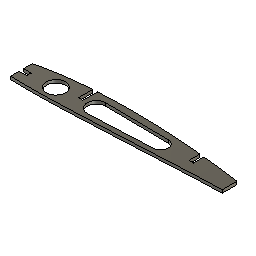
Ala_sola (Autodesk Fusion 360 design; units mm, degrees)
Autodesk Fusion 360 part; units mm, degrees
sketch "Sketch1" plane through (0, 0, -356.8897) normal (0, 0, -1) x (1, 0, 0)
  spline S0 degree 3 poles (-314.9041, -27.3143) (-316.3315, -27.2751) (-317.7488, -27.2348) (-319.1559, -27.1934) (-320.4817, -27.1544) (-321.8989, -27.1118) (-323.4076, -27.0655) (-325.0648, -27.0147) (-326.482, -26.9692) (-327.659, -26.9291) (-329.1964, -26.8766) (-330.6132, -26.8239) (-331.9096, -26.7707) (-333.2219, -26.7169) (-334.6383, -26.653) (-336.1588, -26.579) (-337.3657, -26.5203) (-338.7817, -26.4481) (-340.4069, -26.3625) (-340.9048, -26.3362) (-342.3207, -26.2608) (-344.6545, -26.1362) (-346.3871, -26.0437) (-347.803, -25.9687) (-348.9022, -25.9112) (-350.4533, -25.8302) (-351.8693, -25.7578) (-353.1502, -25.6942) (-354.3709, -25.6336) (-355.7871, -25.5655) (-357.3988, -25.49) (-357.8647, -25.4681) (-358.5729, -25.4351) (-359.5233, -25.3909) (-360.4753, -25.3466) (-361.1835, -25.3136) (-361.6478, -25.2918) (-363.3057, -25.2141) (-364.7219, -25.1456) (-365.8964, -25.0864) (-367.081, -25.0266) (-368.4969, -24.9521) (-370.1441, -24.8628) (-370.6018, -24.8379) (-371.3096, -24.7993) (-372.2678, -24.7469) (-373.1875, -24.6965) (-373.8954, -24.658) (-374.3914, -24.6312) (-375.1751, -24.589) (-375.883, -24.5515) (-376.5152, -24.5187) (-377.2155, -24.4825) (-377.9236, -24.447) (-378.6393, -24.4121) (-379.7568, -24.3578) (-381.1731, -24.2918) (-382.8883, -24.2142) (-383.038, -24.2074) (-383.7462, -24.1755) (-385.0129, -24.1185) (-385.8708, -24.0798) (-386.579, -24.0477) (-387.1375, -24.0222) (-388.4675, -23.9613) (-389.8838, -23.8946) (-391.3864, -23.8221) (-392.4634, -23.7701) (-393.8796, -23.7008) (-395.6349, -23.6141) (-397.743, -23.51) (-399.1591, -23.4403) (-399.8833, -23.405) (-401.4759, -23.3273) (-402.8922, -23.2596) (-404.1321, -23.2021) (-405.6617, -23.1311) (-407.0782, -23.0681) (-408.3815, -23.0132) (-409.7162, -22.957) (-411.1329, -22.901) (-412.6317, -22.8453) (-413.9257, -22.7972) (-415.3427, -22.7469) (-416.8826, -22.6944) (-418.2291, -22.6484) (-419.6462, -22.6016) (-421.1339, -22.5538) (-422.7685, -22.5013) (-424.1858, -22.4583) (-425.3855, -22.4248) (-427.0005, -22.3797) (-428.418, -22.3467) (-429.6379, -22.3256) (-430.9059, -22.3038) (-432.3237, -22.2887) (-433.8912, -22.2804) (-434.4617, -22.2774) (-435.1706, -22.2747) (-436.018, -22.2724) (-436.7269, -22.2704) (-437.4359, -22.2685) (-438.1448, -22.2667) (-438.154, -22.2666) (-438.5085, -22.2655) (-439.2082, -22.2633) (-439.6355, -22.262) (-439.99, -22.2609) (-440.2716, -22.2601) (-441.1017, -22.2579) (-441.8106, -22.2568) (-442.3984, -22.2568) (-443.1776, -22.2569) (-443.8865, -22.2589) (-444.5252, -22.2629) (-445.2443, -22.2674) (-445.9532, -22.2751) (-446.6518, -22.2858) (-448.0829, -22.3077) (-449.5003, -22.3423) (-450.9041, -22.3898) knots 0.19390624 0.19390624 0.19390624 0.19390624 0.20388368 0.20388368 0.20388368 0.21386113 0.21386113 0.21386113 0.22383858 0.22383858 0.22383858 0.23381602 0.23381602 0.23381602 0.24379347 0.24379347 0.24379347 0.25377092 0.25377092 0.25377092 0.26374837 0.26374837 0.26374837 0.27372581 0.27372581 0.27372581 0.28370326 0.28370326 0.28370326 0.29368071 0.29368071 0.29368071 0.29866943 0.29866943 0.29866943 0.30365815 0.30365815 0.30365815 0.3136356 0.3136356 0.3136356 0.32361305 0.32361305 0.32361305 0.32860177 0.32860177 0.32860177 0.3335905 0.3335905 0.3335905 0.33857922 0.33857922 0.33857922 0.34356794 0.34356794 0.34356794 0.35354539 0.35354539 0.35354539 0.35853411 0.35853411 0.35853411 0.36352284 0.36352284 0.36352284 0.37350028 0.37350028 0.37350028 0.38347773 0.38347773 0.38347773 0.39345518 0.39345518 0.39345518 0.40343263 0.40343263 0.40343263 0.41341007 0.41341007 0.41341007 0.42338752 0.42338752 0.42338752 0.43336497 0.43336497 0.43336497 0.44334241 0.44334241 0.44334241 0.45331986 0.45331986 0.45331986 0.46329731 0.46329731 0.46329731 0.47327476 0.47327476 0.47327476 0.47826348 0.47826348 0.47826348 0.4832522 0.4832522 0.4832522 0.48574656 0.48574656 0.48574656 0.48824093 0.48824093 0.48824093 0.49322965 0.49322965 0.49322965 0.49821837 0.49821837 0.49821837 0.5032071 0.5032071 0.5032071 0.51318454 0.51318454 0.51318454 0.51318454
  line L0 (-450.9041, -22.3898) -> (-450.9041, -28.1007)
  line L1 (-450.9041, -28.1007) -> (-445.9041, -28.1007)
  line L2 (-445.9041, -28.1007) -> (-445.9041, -31.1007)
  line L3 (-445.9041, -31.1007) -> (-450.9041, -31.1007)
  line L4 (-450.9041, -31.1007) -> (-450.9041, -36.8116)
  spline S1 degree 3 poles (-450.9041, -36.8116) (-450.2054, -36.9947) (-449.4894, -37.1753) (-448.7562, -37.3534) (-448.0397, -37.5274) (-447.3208, -37.6955) (-446.5992, -37.8577) (-445.2244, -38.1667) (-443.7786, -38.4677) (-442.262, -38.7606) (-440.8373, -39.0357) (-439.3839, -39.297) (-437.9016, -39.5444) (-436.4787, -39.7819) (-435.0193, -40.0079) (-433.5236, -40.2223) (-432.0873, -40.4282) (-430.6235, -40.6232) (-429.1321, -40.8074) (-427.6736, -40.9874) (-426.2064, -41.1548) (-424.7304, -41.3095) (-423.301, -41.4593) (-421.831, -41.6002) (-420.3203, -41.7323) (-418.863, -41.8597) (-417.3909, -41.9773) (-415.9041, -42.0849) knots 0.007053 0.007053 0.007053 0.007053 0.012249 0.012249 0.012249 0.017445 0.017445 0.017445 0.027837 0.027837 0.027837 0.038229 0.038229 0.038229 0.048621 0.048621 0.048621 0.059013 0.059013 0.059013 0.069404 0.069404 0.069404 0.079796 0.079796 0.079796 0.090188 0.090188 0.090188 0.090188
  line L5 (-415.9041, -42.0849) -> (-415.9041, -32.5613)
  line L6 (-415.9041, -32.5613) -> (-412.9041, -32.5613)
  line L7 (-412.9041, -32.5613) -> (-412.9041, -42.2874)
  spline S2 degree 3 poles (-412.9041, -42.2874) (-410.0329, -42.4672) (-407.1159, -42.6103) (-404.1532, -42.7167) (-402.6996, -42.7689) (-401.24, -42.812) (-399.7744, -42.846) (-398.3395, -42.8793) (-396.8794, -42.9043) (-395.3942, -42.9212) (-393.945, -42.9377) (-392.4848, -42.9462) (-391.0135, -42.9467) (-389.5879, -42.9472) (-388.1277, -42.9402) (-386.6327, -42.9256) (-383.6825, -42.8969) (-380.7625, -42.8411) (-377.8728, -42.7582) (-374.9901, -42.6756) (-372.0717, -42.5646) (-369.1177, -42.4253) (-366.2195, -42.2887) (-363.3036, -42.1258) (-360.3698, -41.9367) (-358.7322, -41.8312) (-357.0673, -41.716) (-355.3751, -41.591) (-353.6901, -41.4666) (-352.0263, -41.3363) (-350.3838, -41.2002) (-347.9215, -40.996) (-345.4283, -40.7717) (-342.9041, -40.5272) knots 0.835586 0.835586 0.835586 0.835586 0.856138 0.856138 0.856138 0.866414 0.866414 0.866414 0.87669 0.87669 0.87669 0.886966 0.886966 0.886966 0.897242 0.897242 0.897242 0.917793 0.917793 0.917793 0.938345 0.938345 0.938345 0.958897 0.958897 0.958897 0.97064 0.97064 0.97064 0.982384 0.982384 0.982384 1 1 1 1
  line L8 (-342.9041, -40.5272) -> (-342.9041, -33.3089)
  line L9 (-342.9041, -33.3089) -> (-339.9041, -33.3089)
  line L10 (-339.9041, -33.3089) -> (-339.9041, -40.2289)
  spline S3 degree 3 poles (-339.9041, -40.2289) (-337.8749, -40.0221) (-335.7879, -39.7995) (-333.643, -39.5611) (-331.4764, -39.3202) (-329.3915, -39.0785) (-327.3883, -38.836) (-325.2965, -38.5827) (-323.2143, -38.3187) (-321.1416, -38.044) (-319.1073, -37.7744) (-317.0281, -37.4876) (-314.9041, -37.1837) knots 0.769436 0.769436 0.769436 0.769436 0.784206 0.784206 0.784206 0.798975 0.798975 0.798975 0.813745 0.813745 0.813745 0.828515 0.828515 0.828515 0.828515
  line L11 (-314.9041, -37.1837) -> (-314.9041, -27.3143)
  circle A0 centre (-429.337, -31.1007) radius 6.3498
  arc A1 (-403.3199, -26.4196) -> (-403.9041, -38.7308) centre (-403.9041, -32.5613) ccw
  line L12 (-403.3199, -26.4196) -> (-361.8196, -28.389)
  arc A2 (-361.8196, -38.2288) -> (-361.8196, -28.389) centre (-361.8196, -33.3089) ccw
  line L13 (-361.8196, -38.2288) -> (-403.9041, -38.7308)
extrude "Extrude1" add sketch "Sketch1" against normal blind 2
sketch "Sketch2" plane through (0, 0, -356.8897) normal (0, 0, -1) x (1, 0, 0)
  circle A0 centre (-429.337, -31.1007) radius 6.3498
  arc A1 (-403.3199, -26.4196) -> (-403.9041, -38.7308) centre (-403.9041, -32.5613) ccw
  line L0 (-403.3199, -26.4196) -> (-361.8196, -28.389)
  arc A2 (-361.8196, -38.2288) -> (-361.8196, -28.389) centre (-361.8196, -33.3089) ccw
  line L1 (-361.8196, -38.2288) -> (-403.9041, -38.7308)
  line L2 (-314.9041, -37.1837) -> (-314.9041, -27.3143)
  spline S0 degree 3 poles (-314.9041, -27.3143) (-316.3315, -27.2751) (-317.7488, -27.2348) (-319.1559, -27.1934) (-320.4817, -27.1544) (-321.8989, -27.1118) (-323.4076, -27.0655) (-325.0648, -27.0147) (-326.482, -26.9692) (-327.659, -26.9291) (-329.1964, -26.8766) (-330.6132, -26.8239) (-331.9096, -26.7707) (-333.2219, -26.7169) (-334.6383, -26.653) (-336.1588, -26.579) (-337.3657, -26.5203) (-338.7817, -26.4481) (-340.4069, -26.3625) (-340.9048, -26.3362) (-342.3207, -26.2608) (-344.6545, -26.1362) (-346.3871, -26.0437) (-347.803, -25.9687) (-348.9022, -25.9112) (-350.4533, -25.8302) (-351.8693, -25.7578) (-353.1502, -25.6942) (-354.3709, -25.6336) (-355.7871, -25.5655) (-357.3988, -25.49) (-357.8647, -25.4681) (-358.5729, -25.4351) (-359.5233, -25.3909) (-360.4753, -25.3466) (-361.1835, -25.3136) (-361.6478, -25.2918) (-363.3057, -25.2141) (-364.7219, -25.1456) (-365.8964, -25.0864) (-367.081, -25.0266) (-368.4969, -24.9521) (-370.1441, -24.8628) (-370.6018, -24.8379) (-371.3096, -24.7993) (-372.2678, -24.7469) (-373.1875, -24.6965) (-373.8954, -24.658) (-374.3914, -24.6312) (-375.1751, -24.589) (-375.883, -24.5515) (-376.5152, -24.5187) (-377.2155, -24.4825) (-377.9236, -24.447) (-378.6393, -24.4121) (-379.7568, -24.3578) (-381.1731, -24.2918) (-382.8883, -24.2142) (-383.038, -24.2074) (-383.7462, -24.1755) (-385.0129, -24.1185) (-385.8708, -24.0798) (-386.579, -24.0477) (-387.1375, -24.0222) (-388.4675, -23.9613) (-389.8838, -23.8946) (-391.3864, -23.8221) (-392.4634, -23.7701) (-393.8796, -23.7008) (-395.6349, -23.6141) (-397.743, -23.51) (-399.1591, -23.4403) (-399.8833, -23.405) (-401.4759, -23.3273) (-402.8922, -23.2596) (-404.1321, -23.2021) (-405.6617, -23.1311) (-407.0782, -23.0681) (-408.3815, -23.0132) (-409.7162, -22.957) (-411.1329, -22.901) (-412.6317, -22.8453) (-413.9257, -22.7972) (-415.3427, -22.7469) (-416.8826, -22.6944) (-418.2291, -22.6484) (-419.6462, -22.6016) (-421.1339, -22.5538) (-422.7685, -22.5013) (-424.1858, -22.4583) (-425.3855, -22.4248) (-427.0005, -22.3797) (-428.418, -22.3467) (-429.6379, -22.3256) (-430.9059, -22.3038) (-432.3237, -22.2887) (-433.8912, -22.2804) (-434.4617, -22.2774) (-435.1706, -22.2747) (-436.018, -22.2724) (-436.7269, -22.2704) (-437.4359, -22.2685) (-438.1448, -22.2667) (-438.154, -22.2666) (-438.5085, -22.2655) (-439.2082, -22.2633) (-439.6355, -22.262) (-439.99, -22.2609) (-440.2716, -22.2601) (-441.1017, -22.2579) (-441.8106, -22.2568) (-442.3984, -22.2568) (-443.1776, -22.2569) (-443.8865, -22.2589) (-444.5252, -22.2629) (-445.2443, -22.2674) (-445.9532, -22.2751) (-446.6518, -22.2858) (-448.0829, -22.3077) (-449.5003, -22.3423) (-450.9041, -22.3898) knots 0.19390624 0.19390624 0.19390624 0.19390624 0.20388368 0.20388368 0.20388368 0.21386113 0.21386113 0.21386113 0.22383858 0.22383858 0.22383858 0.23381602 0.23381602 0.23381602 0.24379347 0.24379347 0.24379347 0.25377092 0.25377092 0.25377092 0.26374837 0.26374837 0.26374837 0.27372581 0.27372581 0.27372581 0.28370326 0.28370326 0.28370326 0.29368071 0.29368071 0.29368071 0.29866943 0.29866943 0.29866943 0.30365815 0.30365815 0.30365815 0.3136356 0.3136356 0.3136356 0.32361305 0.32361305 0.32361305 0.32860177 0.32860177 0.32860177 0.3335905 0.3335905 0.3335905 0.33857922 0.33857922 0.33857922 0.34356794 0.34356794 0.34356794 0.35354539 0.35354539 0.35354539 0.35853411 0.35853411 0.35853411 0.36352284 0.36352284 0.36352284 0.37350028 0.37350028 0.37350028 0.38347773 0.38347773 0.38347773 0.39345518 0.39345518 0.39345518 0.40343263 0.40343263 0.40343263 0.41341007 0.41341007 0.41341007 0.42338752 0.42338752 0.42338752 0.43336497 0.43336497 0.43336497 0.44334241 0.44334241 0.44334241 0.45331986 0.45331986 0.45331986 0.46329731 0.46329731 0.46329731 0.47327476 0.47327476 0.47327476 0.47826348 0.47826348 0.47826348 0.4832522 0.4832522 0.4832522 0.48574656 0.48574656 0.48574656 0.48824093 0.48824093 0.48824093 0.49322965 0.49322965 0.49322965 0.49821837 0.49821837 0.49821837 0.5032071 0.5032071 0.5032071 0.51318454 0.51318454 0.51318454 0.51318454
  line L3 (-450.9041, -22.3898) -> (-450.9041, -28.1007)
  line L4 (-450.9041, -28.1007) -> (-445.9041, -28.1007)
  line L5 (-445.9041, -28.1007) -> (-445.9041, -31.1007)
  line L6 (-445.9041, -31.1007) -> (-450.9041, -31.1007)
  line L7 (-450.9041, -31.1007) -> (-450.9041, -36.8116)
  spline S1 degree 3 poles (-450.9041, -36.8116) (-450.2054, -36.9947) (-449.4894, -37.1753) (-448.7562, -37.3534) (-448.0397, -37.5274) (-447.3208, -37.6955) (-446.5992, -37.8577) (-445.2244, -38.1667) (-443.7786, -38.4677) (-442.262, -38.7606) (-440.8373, -39.0357) (-439.3839, -39.297) (-437.9016, -39.5444) (-436.4787, -39.7819) (-435.0193, -40.0079) (-433.5236, -40.2223) (-432.0873, -40.4282) (-430.6235, -40.6232) (-429.1321, -40.8074) (-427.6736, -40.9874) (-426.2064, -41.1548) (-424.7304, -41.3095) (-423.301, -41.4593) (-421.831, -41.6002) (-420.3203, -41.7323) (-418.863, -41.8597) (-417.3909, -41.9773) (-415.9041, -42.0849) knots 0.007053 0.007053 0.007053 0.007053 0.012249 0.012249 0.012249 0.017445 0.017445 0.017445 0.027837 0.027837 0.027837 0.038229 0.038229 0.038229 0.048621 0.048621 0.048621 0.059013 0.059013 0.059013 0.069404 0.069404 0.069404 0.079796 0.079796 0.079796 0.090188 0.090188 0.090188 0.090188
  line L8 (-415.9041, -42.0849) -> (-415.9041, -32.5613)
  line L9 (-415.9041, -32.5613) -> (-412.9041, -32.5613)
  line L10 (-412.9041, -32.5613) -> (-412.9041, -42.2874)
  spline S2 degree 3 poles (-412.9041, -42.2874) (-410.0329, -42.4672) (-407.1159, -42.6103) (-404.1532, -42.7167) (-402.6996, -42.7689) (-401.24, -42.812) (-399.7744, -42.846) (-398.3395, -42.8793) (-396.8794, -42.9043) (-395.3942, -42.9212) (-393.945, -42.9377) (-392.4848, -42.9462) (-391.0135, -42.9467) (-389.5879, -42.9472) (-388.1277, -42.9402) (-386.6327, -42.9256) (-383.6825, -42.8969) (-380.7625, -42.8411) (-377.8728, -42.7582) (-374.9901, -42.6756) (-372.0717, -42.5646) (-369.1177, -42.4253) (-366.2195, -42.2887) (-363.3036, -42.1258) (-360.3698, -41.9367) (-358.7322, -41.8312) (-357.0673, -41.716) (-355.3751, -41.591) (-353.6901, -41.4666) (-352.0263, -41.3363) (-350.3838, -41.2002) (-347.9215, -40.996) (-345.4283, -40.7717) (-342.9041, -40.5272) knots 0.835586 0.835586 0.835586 0.835586 0.856138 0.856138 0.856138 0.866414 0.866414 0.866414 0.87669 0.87669 0.87669 0.886966 0.886966 0.886966 0.897242 0.897242 0.897242 0.917793 0.917793 0.917793 0.938345 0.938345 0.938345 0.958897 0.958897 0.958897 0.97064 0.97064 0.97064 0.982384 0.982384 0.982384 1 1 1 1
  line L11 (-342.9041, -40.5272) -> (-342.9041, -33.3089)
  line L12 (-342.9041, -33.3089) -> (-339.9041, -33.3089)
  line L13 (-339.9041, -33.3089) -> (-339.9041, -40.2289)
  spline S3 degree 3 poles (-339.9041, -40.2289) (-337.8749, -40.0221) (-335.7879, -39.7995) (-333.643, -39.5611) (-331.4764, -39.3202) (-329.3915, -39.0785) (-327.3883, -38.836) (-325.2965, -38.5827) (-323.2143, -38.3187) (-321.1416, -38.044) (-319.1073, -37.7744) (-317.0281, -37.4876) (-314.9041, -37.1837) knots 0.769436 0.769436 0.769436 0.769436 0.784206 0.784206 0.784206 0.798975 0.798975 0.798975 0.813745 0.813745 0.813745 0.828515 0.828515 0.828515 0.828515
  line L14 (-412.9041, -32.5613) -> (-415.9041, -32.5613)
  line L15 (-415.9041, -32.5613) -> (-415.9041, -47.9137)
  line L16 (-415.9041, -47.9137) -> (-412.9041, -47.9137)
  line L17 (-412.9041, -47.9137) -> (-412.9041, -32.5613)
  line L18 (-342.9041, -33.3089) -> (-339.9041, -33.3089)
  line L19 (-339.9041, -33.3089) -> (-339.9041, -44.8961)
  line L20 (-339.9041, -44.8961) -> (-342.9041, -44.8961)
  line L21 (-342.9041, -44.8961) -> (-342.9041, -33.3089)
  line L22 (-445.9041, -28.1007) -> (-458.839, -28.1007)
  line L23 (-458.839, -28.1007) -> (-458.839, -31.1007)
  line L24 (-458.839, -31.1007) -> (-445.9041, -31.1007)
  line L25 (-445.9041, -31.1007) -> (-445.9041, -28.1007)
  circle A3 centre (-429.337, -31.1007) radius 6.3498
  constraint horizontal L14
  constraint vertical L15
  constraint horizontal L16
  constraint vertical L17
  constraint coincident L9.end L10.start
  constraint horizontal L18
  constraint vertical L19
  constraint horizontal L20
  constraint vertical L21
  constraint coincident L11.end L12.start
  constraint coincident L8.end L9.start
  constraint horizontal L22
  constraint vertical L23
  constraint horizontal L24
  constraint vertical L25
  constraint coincident L4.end L5.start
sketch "Sketch3" plane through (0, 0, -356.8897) normal (0, 0, -1) x (1, 0, 0)
  circle A0 centre (-429.337, -31.1007) radius 6.3498
  arc A1 (-403.3199, -26.4196) -> (-403.9041, -38.7308) centre (-403.9041, -32.5613) ccw
  line L0 (-403.3199, -26.4196) -> (-361.8196, -28.389)
  arc A2 (-361.8196, -38.2288) -> (-361.8196, -28.389) centre (-361.8196, -33.3089) ccw
  line L1 (-361.8196, -38.2288) -> (-403.9041, -38.7308)
  line L2 (-314.9041, -37.1837) -> (-314.9041, -27.3143)
  spline S0 degree 3 poles (-314.9041, -27.3143) (-316.3315, -27.2751) (-317.7488, -27.2348) (-319.1559, -27.1934) (-320.4817, -27.1544) (-321.8989, -27.1118) (-323.4076, -27.0655) (-325.0648, -27.0147) (-326.482, -26.9692) (-327.659, -26.9291) (-329.1964, -26.8766) (-330.6132, -26.8239) (-331.9096, -26.7707) (-333.2219, -26.7169) (-334.6383, -26.653) (-336.1588, -26.579) (-337.3657, -26.5203) (-338.7817, -26.4481) (-340.4069, -26.3625) (-340.9048, -26.3362) (-342.3207, -26.2608) (-344.6545, -26.1362) (-346.3871, -26.0437) (-347.803, -25.9687) (-348.9022, -25.9112) (-350.4533, -25.8302) (-351.8693, -25.7578) (-353.1502, -25.6942) (-354.3709, -25.6336) (-355.7871, -25.5655) (-357.3988, -25.49) (-357.8647, -25.4681) (-358.5729, -25.4351) (-359.5233, -25.3909) (-360.4753, -25.3466) (-361.1835, -25.3136) (-361.6478, -25.2918) (-363.3057, -25.2141) (-364.7219, -25.1456) (-365.8964, -25.0864) (-367.081, -25.0266) (-368.4969, -24.9521) (-370.1441, -24.8628) (-370.6018, -24.8379) (-371.3096, -24.7993) (-372.2678, -24.7469) (-373.1875, -24.6965) (-373.8954, -24.658) (-374.3914, -24.6312) (-375.1751, -24.589) (-375.883, -24.5515) (-376.5152, -24.5187) (-377.2155, -24.4825) (-377.9236, -24.447) (-378.6393, -24.4121) (-379.7568, -24.3578) (-381.1731, -24.2918) (-382.8883, -24.2142) (-383.038, -24.2074) (-383.7462, -24.1755) (-385.0129, -24.1185) (-385.8708, -24.0798) (-386.579, -24.0477) (-387.1375, -24.0222) (-388.4675, -23.9613) (-389.8838, -23.8946) (-391.3864, -23.8221) (-392.4634, -23.7701) (-393.8796, -23.7008) (-395.6349, -23.6141) (-397.743, -23.51) (-399.1591, -23.4403) (-399.8833, -23.405) (-401.4759, -23.3273) (-402.8922, -23.2596) (-404.1321, -23.2021) (-405.6617, -23.1311) (-407.0782, -23.0681) (-408.3815, -23.0132) (-409.7162, -22.957) (-411.1329, -22.901) (-412.6317, -22.8453) (-413.9257, -22.7972) (-415.3427, -22.7469) (-416.8826, -22.6944) (-418.2291, -22.6484) (-419.6462, -22.6016) (-421.1339, -22.5538) (-422.7685, -22.5013) (-424.1858, -22.4583) (-425.3855, -22.4248) (-427.0005, -22.3797) (-428.418, -22.3467) (-429.6379, -22.3256) (-430.9059, -22.3038) (-432.3237, -22.2887) (-433.8912, -22.2804) (-434.4617, -22.2774) (-435.1706, -22.2747) (-436.018, -22.2724) (-436.7269, -22.2704) (-437.4359, -22.2685) (-438.1448, -22.2667) (-438.154, -22.2666) (-438.5085, -22.2655) (-439.2082, -22.2633) (-439.6355, -22.262) (-439.99, -22.2609) (-440.2716, -22.2601) (-441.1017, -22.2579) (-441.8106, -22.2568) (-442.3984, -22.2568) (-443.1776, -22.2569) (-443.8865, -22.2589) (-444.5252, -22.2629) (-445.2443, -22.2674) (-445.9532, -22.2751) (-446.6518, -22.2858) (-448.0829, -22.3077) (-449.5003, -22.3423) (-450.9041, -22.3898) knots 0.19390624 0.19390624 0.19390624 0.19390624 0.20388368 0.20388368 0.20388368 0.21386113 0.21386113 0.21386113 0.22383858 0.22383858 0.22383858 0.23381602 0.23381602 0.23381602 0.24379347 0.24379347 0.24379347 0.25377092 0.25377092 0.25377092 0.26374837 0.26374837 0.26374837 0.27372581 0.27372581 0.27372581 0.28370326 0.28370326 0.28370326 0.29368071 0.29368071 0.29368071 0.29866943 0.29866943 0.29866943 0.30365815 0.30365815 0.30365815 0.3136356 0.3136356 0.3136356 0.32361305 0.32361305 0.32361305 0.32860177 0.32860177 0.32860177 0.3335905 0.3335905 0.3335905 0.33857922 0.33857922 0.33857922 0.34356794 0.34356794 0.34356794 0.35354539 0.35354539 0.35354539 0.35853411 0.35853411 0.35853411 0.36352284 0.36352284 0.36352284 0.37350028 0.37350028 0.37350028 0.38347773 0.38347773 0.38347773 0.39345518 0.39345518 0.39345518 0.40343263 0.40343263 0.40343263 0.41341007 0.41341007 0.41341007 0.42338752 0.42338752 0.42338752 0.43336497 0.43336497 0.43336497 0.44334241 0.44334241 0.44334241 0.45331986 0.45331986 0.45331986 0.46329731 0.46329731 0.46329731 0.47327476 0.47327476 0.47327476 0.47826348 0.47826348 0.47826348 0.4832522 0.4832522 0.4832522 0.48574656 0.48574656 0.48574656 0.48824093 0.48824093 0.48824093 0.49322965 0.49322965 0.49322965 0.49821837 0.49821837 0.49821837 0.5032071 0.5032071 0.5032071 0.51318454 0.51318454 0.51318454 0.51318454
  line L3 (-450.9041, -22.3898) -> (-450.9041, -28.1007)
  line L4 (-450.9041, -28.1007) -> (-445.9041, -28.1007)
  line L5 (-445.9041, -28.1007) -> (-445.9041, -31.1007)
  line L6 (-445.9041, -31.1007) -> (-450.9041, -31.1007)
  line L7 (-450.9041, -31.1007) -> (-450.9041, -36.8116)
  spline S1 degree 3 poles (-450.9041, -36.8116) (-450.2054, -36.9947) (-449.4894, -37.1753) (-448.7562, -37.3534) (-448.0397, -37.5274) (-447.3208, -37.6955) (-446.5992, -37.8577) (-445.2244, -38.1667) (-443.7786, -38.4677) (-442.262, -38.7606) (-440.8373, -39.0357) (-439.3839, -39.297) (-437.9016, -39.5444) (-436.4787, -39.7819) (-435.0193, -40.0079) (-433.5236, -40.2223) (-432.0873, -40.4282) (-430.6235, -40.6232) (-429.1321, -40.8074) (-427.6736, -40.9874) (-426.2064, -41.1548) (-424.7304, -41.3095) (-423.301, -41.4593) (-421.831, -41.6002) (-420.3203, -41.7323) (-418.863, -41.8597) (-417.3909, -41.9773) (-415.9041, -42.0849) knots 0.007053 0.007053 0.007053 0.007053 0.012249 0.012249 0.012249 0.017445 0.017445 0.017445 0.027837 0.027837 0.027837 0.038229 0.038229 0.038229 0.048621 0.048621 0.048621 0.059013 0.059013 0.059013 0.069404 0.069404 0.069404 0.079796 0.079796 0.079796 0.090188 0.090188 0.090188 0.090188
  line L8 (-415.9041, -42.0849) -> (-415.9041, -32.5613)
  line L9 (-415.9041, -32.5613) -> (-412.9041, -32.5613)
  line L10 (-412.9041, -32.5613) -> (-412.9041, -42.2874)
  spline S2 degree 3 poles (-412.9041, -42.2874) (-410.0329, -42.4672) (-407.1159, -42.6103) (-404.1532, -42.7167) (-402.6996, -42.7689) (-401.24, -42.812) (-399.7744, -42.846) (-398.3395, -42.8793) (-396.8794, -42.9043) (-395.3942, -42.9212) (-393.945, -42.9377) (-392.4848, -42.9462) (-391.0135, -42.9467) (-389.5879, -42.9472) (-388.1277, -42.9402) (-386.6327, -42.9256) (-383.6825, -42.8969) (-380.7625, -42.8411) (-377.8728, -42.7582) (-374.9901, -42.6756) (-372.0717, -42.5646) (-369.1177, -42.4253) (-366.2195, -42.2887) (-363.3036, -42.1258) (-360.3698, -41.9367) (-358.7322, -41.8312) (-357.0673, -41.716) (-355.3751, -41.591) (-353.6901, -41.4666) (-352.0263, -41.3363) (-350.3838, -41.2002) (-347.9215, -40.996) (-345.4283, -40.7717) (-342.9041, -40.5272) knots 0.835586 0.835586 0.835586 0.835586 0.856138 0.856138 0.856138 0.866414 0.866414 0.866414 0.87669 0.87669 0.87669 0.886966 0.886966 0.886966 0.897242 0.897242 0.897242 0.917793 0.917793 0.917793 0.938345 0.938345 0.938345 0.958897 0.958897 0.958897 0.97064 0.97064 0.97064 0.982384 0.982384 0.982384 1 1 1 1
  line L11 (-342.9041, -40.5272) -> (-342.9041, -33.3089)
  line L12 (-342.9041, -33.3089) -> (-339.9041, -33.3089)
  line L13 (-339.9041, -33.3089) -> (-339.9041, -40.2289)
  spline S3 degree 3 poles (-339.9041, -40.2289) (-337.8749, -40.0221) (-335.7879, -39.7995) (-333.643, -39.5611) (-331.4764, -39.3202) (-329.3915, -39.0785) (-327.3883, -38.836) (-325.2965, -38.5827) (-323.2143, -38.3187) (-321.1416, -38.044) (-319.1073, -37.7744) (-317.0281, -37.4876) (-314.9041, -37.1837) knots 0.769436 0.769436 0.769436 0.769436 0.784206 0.784206 0.784206 0.798975 0.798975 0.798975 0.813745 0.813745 0.813745 0.828515 0.828515 0.828515 0.828515
  line L14 (-449.9041, -27.1007) -> (-444.9041, -27.1007)
  line L15 (-444.9041, -27.1007) -> (-444.9041, -32.1007)
  line L16 (-444.9041, -32.1007) -> (-449.9041, -32.1007)
  line L17 (-449.9041, -32.1007) -> (-449.9041, -36.0372)
  spline S4 degree 3 poles (-449.9041, -36.0372) (-449.4501, -36.153) (-448.9887, -36.2678) (-448.5202, -36.3817) (-447.8093, -36.5543) (-447.0959, -36.7211) (-446.3799, -36.8821) knots 0.008903 0.008903 0.008903 0.008903 0.012249 0.012249 0.012249 0.017445 0.017445 0.017445 0.017445
  spline S5 degree 3 poles (-446.3799, -36.8821) (-445.0159, -37.1887) (-443.5799, -37.4876) (-442.0724, -37.7787) (-440.6563, -38.0522) (-439.2112, -38.312) (-437.737, -38.558) (-436.322, -38.7942) (-434.8702, -39.019) (-433.3817, -39.2324) (-431.9521, -39.4374) (-430.4947, -39.6315) (-429.0096, -39.8149) (-427.5573, -39.9942) (-426.0961, -40.1609) (-424.6262, -40.3149) (-423.2028, -40.4641) (-421.7385, -40.6045) (-420.2332, -40.7361) knots 0.017445 0.017445 0.017445 0.017445 0.027837 0.027837 0.027837 0.038229 0.038229 0.038229 0.048621 0.048621 0.048621 0.059013 0.059013 0.059013 0.069404 0.069404 0.069404 0.079796 0.079796 0.079796 0.079796
  spline S6 degree 3 poles (-420.2332, -40.7361) (-419.132, -40.8324) (-418.0223, -40.923) (-416.9041, -41.008) knots 0.079796 0.079796 0.079796 0.079796 0.087676 0.087676 0.087676 0.087676
  line L18 (-416.9041, -41.008) -> (-416.9041, -31.5613)
  line L19 (-416.9041, -31.5613) -> (-411.9041, -31.5613)
  line L20 (-411.9041, -31.5613) -> (-411.9041, -41.3466)
  spline S7 degree 3 poles (-411.9041, -41.3466) (-409.345, -41.4992) (-406.7494, -41.6228) (-404.1173, -41.7173) (-402.668, -41.7694) (-401.2126, -41.8124) (-399.7512, -41.8463) (-398.3204, -41.8794) (-396.8643, -41.9045) (-395.3828, -41.9213) knots 0.837827 0.837827 0.837827 0.837827 0.856138 0.856138 0.856138 0.866414 0.866414 0.866414 0.87669 0.87669 0.87669 0.87669
  spline S8 degree 3 poles (-395.3828, -41.9213) (-393.9374, -41.9377) (-392.4808, -41.9462) (-391.0131, -41.9467) (-389.5911, -41.9472) (-388.1342, -41.9402) (-386.6425, -41.9257) (-383.6984, -41.897) (-380.7848, -41.8413) (-377.9015, -41.7587) (-375.0251, -41.6762) (-372.1128, -41.5654) (-369.1648, -41.4264) (-366.2725, -41.2901) (-363.3622, -41.1275) (-360.4341, -40.9388) (-358.7997, -40.8335) (-357.1379, -40.7185) (-355.4488, -40.5937) (-353.7666, -40.4696) (-352.1058, -40.3395) (-350.4664, -40.2036) (-348.303, -40.0242) (-346.1156, -39.8293) (-343.9041, -39.6187) knots 0.87669 0.87669 0.87669 0.87669 0.886966 0.886966 0.886966 0.897242 0.897242 0.897242 0.917793 0.917793 0.917793 0.938345 0.938345 0.938345 0.958897 0.958897 0.958897 0.97064 0.97064 0.97064 0.982384 0.982384 0.982384 0.997891 0.997891 0.997891 0.997891
  line L21 (-343.9041, -39.6187) -> (-343.9041, -32.3089)
  line L22 (-343.9041, -32.3089) -> (-338.9041, -32.3089)
  line L23 (-338.9041, -32.3089) -> (-338.9041, -39.1209)
  spline S9 degree 3 poles (-338.9041, -39.1209) (-337.2262, -38.9469) (-335.5093, -38.7624) (-333.7535, -38.5672) (-331.5899, -38.3267) (-329.5082, -38.0853) (-327.5085, -37.8432) (-325.4204, -37.5904) (-323.3419, -37.3269) (-321.273, -37.0527) (-319.517, -36.8199) (-317.7274, -36.5744) (-315.9041, -36.316) knots 0.772098 0.772098 0.772098 0.772098 0.784206 0.784206 0.784206 0.798975 0.798975 0.798975 0.813745 0.813745 0.813745 0.826516 0.826516 0.826516 0.826516
  line L24 (-315.9041, -36.316) -> (-315.9041, -28.287)
  spline S10 degree 3 poles (-315.9041, -28.287) (-317.0039, -28.2563) (-318.0976, -28.225) (-319.1853, -28.193) knots 0.196175 0.196175 0.196175 0.196175 0.203884 0.203884 0.203884 0.203884
  spline S11 degree 3 poles (-319.1853, -28.193) (-320.5116, -28.154) (-321.9292, -28.1113) (-323.4382, -28.065) (-325.0963, -28.0142) (-326.5145, -27.9687) (-327.693, -27.9285) (-329.2324, -27.876) (-330.6515, -27.8231) (-331.9506, -27.7698) (-333.2658, -27.7159) (-334.6847, -27.6519) (-336.2074, -27.5778) (-337.4161, -27.519) (-338.8333, -27.4468) (-340.4596, -27.3611) (-340.9585, -27.3348) (-342.3739, -27.2594) (-344.7079, -27.1348) (-346.4402, -27.0423) (-347.8558, -26.9673) (-348.9544, -26.9099) (-350.5048, -26.8288) (-351.92, -26.7565) (-353.1998, -26.693) (-354.4192, -26.6324) (-355.8346, -26.5644) (-357.4457, -26.4889) knots 0.203884 0.203884 0.203884 0.203884 0.213861 0.213861 0.213861 0.223839 0.223839 0.223839 0.233816 0.233816 0.233816 0.243793 0.243793 0.243793 0.253771 0.253771 0.253771 0.263748 0.263748 0.263748 0.273726 0.273726 0.273726 0.283703 0.283703 0.283703 0.293681 0.293681 0.293681 0.293681
  spline S12 degree 3 poles (-357.4457, -26.4889) (-357.9113, -26.467) (-358.6194, -26.434) (-359.5698, -26.3898) (-360.5218, -26.3456) (-361.23, -26.3125) (-361.6947, -26.2907) knots 0.293681 0.293681 0.293681 0.293681 0.298669 0.298669 0.298669 0.303658 0.303658 0.303658 0.303658
  spline S13 degree 3 poles (-361.6947, -26.2907) (-363.3533, -26.2129) (-364.7706, -26.1444) (-365.9468, -26.0851) (-367.1331, -26.0253) (-368.5502, -25.9507) (-370.1983, -25.8613) knots 0.303658 0.303658 0.303658 0.303658 0.313636 0.313636 0.313636 0.323613 0.323613 0.323613 0.323613
  spline S14 degree 3 poles (-370.1983, -25.8613) (-370.6563, -25.8364) (-371.3642, -25.7978) (-372.3224, -25.7454) (-373.242, -25.6951) (-373.9497, -25.6565) (-374.4453, -25.6298) knots 0.323613 0.323613 0.323613 0.323613 0.328602 0.328602 0.328602 0.33359 0.33359 0.33359 0.33359
  spline S15 degree 3 poles (-374.4453, -25.6298) (-375.2284, -25.5876) (-375.9356, -25.5501) (-376.5669, -25.5174) knots 0.33359 0.33359 0.33359 0.33359 0.338579 0.338579 0.338579 0.338579
  spline S16 degree 3 poles (-376.5669, -25.5174) (-377.2662, -25.4812) (-377.9732, -25.4457) (-378.6879, -25.411) knots 0.338579 0.338579 0.338579 0.338579 0.343568 0.343568 0.343568 0.343568
  spline S17 degree 3 poles (-378.6879, -25.411) (-379.8036, -25.3567) (-381.219, -25.2907) (-382.9335, -25.2132) knots 0.343568 0.343568 0.343568 0.343568 0.353545 0.353545 0.353545 0.353545
  spline S18 degree 3 poles (-382.9335, -25.2132) (-383.0827, -25.2064) (-383.7912, -25.1745) (-385.0579, -25.1174) (-385.916, -25.0788) (-386.6244, -25.0467) (-387.1832, -25.0211) knots 0.353545 0.353545 0.353545 0.353545 0.358534 0.358534 0.358534 0.363523 0.363523 0.363523 0.363523
  spline S19 degree 3 poles (-387.1832, -25.0211) (-388.5141, -24.9602) (-389.9312, -24.8935) (-391.4346, -24.8209) knots 0.363523 0.363523 0.363523 0.363523 0.3735 0.3735 0.3735 0.3735
  spline S20 degree 3 poles (-391.4346, -24.8209) (-392.5122, -24.7689) (-393.9287, -24.6996) (-395.6842, -24.6129) (-397.7922, -24.5088) (-399.2084, -24.4391) (-399.9321, -24.4038) knots 0.3735 0.3735 0.3735 0.3735 0.383478 0.383478 0.383478 0.393455 0.393455 0.393455 0.393455
  spline S21 degree 3 poles (-399.9321, -24.4038) (-401.5241, -24.3261) (-402.9396, -24.2585) (-404.1784, -24.201) (-405.7069, -24.1301) (-407.122, -24.0672) (-408.4235, -24.0123) (-409.7564, -23.9561) (-411.1716, -23.9002) (-412.6689, -23.8446) (-413.9617, -23.7965) (-415.3776, -23.7463) (-416.9167, -23.6938) knots 0.393455 0.393455 0.393455 0.393455 0.403433 0.403433 0.403433 0.41341 0.41341 0.41341 0.423388 0.423388 0.423388 0.433365 0.433365 0.433365 0.433365
  spline S22 degree 3 poles (-416.9167, -23.6938) (-418.2624, -23.6479) (-419.6789, -23.601) (-421.166, -23.5533) (-422.7996, -23.5008) (-424.2156, -23.4578) (-425.4134, -23.4244) (-427.0257, -23.3794) (-428.44, -23.3464) (-429.6552, -23.3255) (-430.9182, -23.3037) (-432.3322, -23.2886) (-433.8965, -23.2804) knots 0.433365 0.433365 0.433365 0.433365 0.443342 0.443342 0.443342 0.45332 0.45332 0.45332 0.463297 0.463297 0.463297 0.473275 0.473275 0.473275 0.473275
  spline S23 degree 3 poles (-433.8965, -23.2804) (-434.4657, -23.2774) (-435.1739, -23.2747) (-436.0208, -23.2724) (-436.7297, -23.2704) (-437.4386, -23.2685) (-438.1475, -23.2666) (-438.1547, -23.2666) (-438.1919, -23.2665) (-438.2707, -23.2663) (-438.4298, -23.2658) (-438.7433, -23.2648) (-439.2113, -23.2633) knots 0.473275 0.473275 0.473275 0.473275 0.478263 0.478263 0.478263 0.483252 0.483252 0.483252 0.484078 0.484078 0.484078 0.485747 0.485747 0.485747 0.485747
  spline S24 degree 3 poles (-439.2113, -23.2633) (-439.6386, -23.2619) (-439.9929, -23.2609) (-440.2743, -23.2601) (-441.1037, -23.2579) (-441.8119, -23.2568) (-442.3983, -23.2568) (-443.1758, -23.2569) (-443.8828, -23.2589) (-444.5189, -23.2629) (-445.2351, -23.2674) (-445.9409, -23.275) (-446.6365, -23.2856) (-447.7339, -23.3024) (-448.8231, -23.3268) (-449.9041, -23.3586) knots 0.485747 0.485747 0.485747 0.485747 0.488241 0.488241 0.488241 0.49323 0.49323 0.49323 0.498218 0.498218 0.498218 0.503207 0.503207 0.503207 0.51089 0.51089 0.51089 0.51089
  line L25 (-449.9041, -23.3586) -> (-449.9041, -27.1007)
  constraint parallel L4 L14
  constraint parallel L5 L15
  constraint parallel L6 L16
  constraint parallel L7 L17
  constraint parallel L8 L18
  constraint parallel L9 L19
  constraint parallel L10 L20
  constraint parallel L11 L21
  constraint parallel L12 L22
  constraint parallel L13 L23
  constraint parallel L2 L24
  constraint parallel L3 L25
extrude "Extrude2" [suppressed]
named bodies: "Original"
